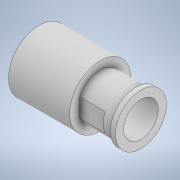
# Autodesk Inventor part: 2
Saved by Autodesk Inventor 2020 (Build 240168000, 168)
## iProperties
Created: 2022-04-06
Part Number: 2
Material: Типовые
Document SubType Name: Modeling
Designer: User
Density: 1 g/cm^3
Appearance: По умолчанию
Author: User
Autodesk Inventor part; units mm, degrees
ref_plane "YZ Plane" through (0, 0, 0) normal (1, 0, 0) x (0, 1, 0)
ref_plane "XZ Plane" through (0, 0, 0) normal (0, 1, 0) x (-1, 0, 0)
ref_plane "XY Plane" through (0, 0, 0) normal (0, 0, 1) x (1, 0, 0)
sketch "Эскиз1" plane through (0, 0, 0) normal (0, 0, 1) x (1, 0, 0)
  line L0 (0, 0) -> (100, 0)
  line L1 (0, 0) -> (0, 30)
  line L2 (0, 30) -> (60, 30)
  line L3 (60, 30) -> (60, 0)
  line L4 (100, 0) -> (100, 25)
  line L5 (100, 25) -> (95, 25)
  line L6 (95, 25) -> (95, 22)
  line L7 (95, 22) -> (25, 22)
  line L8 (25, 22) -> (25, 25)
  line L9 (25, 25) -> (20, 25)
  line L10 (20, 25) -> (20, 0)
  line L11 (0, 20) -> (10, 20)
  line L12 (10, 20) -> (10, 17)
  line L13 (10, 17) -> (20, 17)
  line L14 (30, 22) -> (30, 17)
  line L15 (30, 17) -> (100, 17)
  point P0 (60, 22)
  dimension "d0" = 100
  dimension "d1" = 30
  dimension "d2" = 60
  dimension "d3" = 25
  dimension "d4" = 5
  dimension "d5" = 3
  dimension "d6" = 70
  dimension "d7" = 3
  dimension "d8" = 5
  dimension "d9" = 10
  dimension "d10" = 3
  dimension "d11" = 8
  dimension "d13" = 70
  dimension "d14" = 8
  dimension "d15" = 40
  dimension "d16" = 5
  constraints: 32 end point, 10 perpendicular, 8 point on line, 2 vertical, 1 horizontal, 1 parallel
  measures "d0" distance of L0.start L0.end
  measures "d1" distance of L0.start L1.end
  measures "d2" distance of L1.end L2.end
  measures "d3" distance of L0.end L4.end
  measures "d4" distance of L4.end L5.end
  measures "d5" distance of L5.end L6.end
  measures "d6" distance of L6.end L7.end
  measures "d7" distance of L7.end L8.end
  measures "d8" distance of L8.end L9.end
  measures "d9" distance of L11.start L11.end
  measures "d10" distance of L11.end L12.end
  measures "d11" distance between parallel lines of L9 L13
  measures "d13" distance between parallel lines of L14 L4
  measures "d14" distance between parallel lines of L15 L5
  measures "d15" distance from line of point (60, 22) L4
  measures "d16" distance from line of point (60, 22) L15
revolve "Вращение1" add sketch "Эскиз1" angle 360 about axis through (0, 0, 0) along (1, 0, 0)
revolve "Вращение2" cut sketch "Эскиз1" angle 360 about axis through (0, 0, 0) along (1, 0, 0) contours L1 L11 L12 L13 L10 L0 | L10 L9 L8 L7 L14 L15 L3 L0 | L3 L15 L4 L0
sketch "Эскиз2" plane through (0, 0, 0) normal (0, 1, 0) x (-1, 0, 0)
  line L0 (-60, 22) -> (-60, -22) projected
  line L1 (-60, -22) -> (-85, -22)
  line L2 (-60, -22) -> (-95, -22) projected
  line L3 (-85, -22) -> (-85, -20)
  line L4 (-85, -20) -> (-60, -20)
  line L5 (-100, -17) -> (-30, -17) projected
  line L6 (-60, -20) -> (-60, -22)
  line L7 (-60, 22) -> (-85, 22)
  line L8 (-60, 22) -> (-95, 22) projected
  line L9 (-85, 22) -> (-85, 20)
  line L10 (-85, 20) -> (-60, 20)
  point P0 (0, 0)
  dimension "d18" = 25
  dimension "d19" = 2
  dimension "d20" = 25
  dimension "d21" = 2
  constraints: 14 end point, 3 perpendicular, 3 point on line, 1 parallel, 1 vertical
  measures "d18" distance of L0.end L1.end
  measures "d19" distance of L1.end L3.end
  measures "d20" distance of L0.start L7.end
  measures "d21" distance of L7.end L9.end
extrude "Выдавливание1" cut sketch "Эскиз2" along normal through all both and the other way through all
